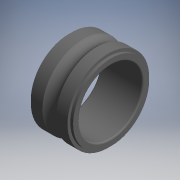
# Autodesk Inventor part: MR126ZZ Inner Ring
Saved by Autodesk Inventor 2017.3 (Build 213256000, 256)
## iProperties
Part Number: MR126ZZ Inner Ring
Material: Generic
Catalog Web Link: www.cadenas.de
Description: shielde_type_zz_zzs_IR-
Vendor: NSK_RB
Document SubType Name: Modeling
Designer: partserver
Manufacturer: NSK_RB
Mass: 0.0656368 g
Surface Area: 2.08449 cm^2
Volume: 0.0656368 cm^3
Density: 1 g/cm^3
Appearance: PSOLRGB-128-128-128
Category: PARTsolutions
Company: NSK_RB
Title: MR126ZZ Inner Ring
Author: Cadenas PARTsolutions
PSOL_IDENT_0: {$CADENAS_DATA\23d-libs\nsk_rb\roller_bearings\deep_groove_bb\exstra_small_miniatur_bb\metric_design
PSOL_IDENT_1: \shielded_type_zz_zzs_ir.prj},193 {VTYP=3D},{NB=MR126ZZ Inner Ring},{LINA=MR126ZZ Inner Ring},{NN=sh
PSOL_IDENT_2: ielde_type_zz_zzs_IR},{DATE=16.07.2021 00:25:30},{GEOMDATE=04.01.2008 00:00:00},{VERSION=},{LINEID=5
PSOL_IDENT_3: 90},{WBVAR=},{WBNUMERIC=}  {NB=MR126ZZ Inner Ring},{LINA=MR126ZZ Inner Ring},{KT=DUMMY},{IDNR=},{STA
PSOL_IDENT_4: N=Standard},{ORDER=MR126ZZ},{SD=6.0},{X=6.0},{DI1=7.73},{DI2=7.20},{SDE1=10.19},{SDE2=10.90},{D=12},
PSOL_IDENT_5: {DD=12},{B=0.0},{B1=4.0},{R=0.00},{R1=0.15},{CR1=715},{COR1=292},{CR2=73},{COR2=30.0},{LG=43000},{LO=
PSOL_IDENT_6: 50000},{DA=0.0},{DB=7.2},{DA1=0.0},{DB1=10.9},{RA=0.00},{RB=0.15},{MASS=1.74},{SC=1},{N=12}
NB: MR126ZZ Inner Ring
NN: shielde_type_zz_zzs_IR
NBSYN: $ORDER. Inner Ring
LINA: MR126ZZ Inner Ring
CATALOG: NSK Rolling Bearing
STAN: Standard
ORDER: MR126ZZ
SD: 6
X: 6
DI1: 7.73
DI2: 7.2
SDE1: 10.19
SDE2: 10.9
D: 12
DD: 12
B: 0
B1: 4
R: 0
R1: 0.15
CR1: 715
COR1: 292
CR2: 73
COR2: 30
LG: 43000
LO: 50000
DA: 0
DB: 7.2
DA1: 0
DB1: 10.9
RA: 0
RB: 0.15
MASS: 1.74
SC: 1
SUPPLIER: NSK_RB
ARTICLENO: MR126ZZ Inner Ring
BOMINFO: MR126ZZ Inner Ring
CREATOR: CADENAS GmbH
Autodesk Inventor part; units mm, degrees
sketch "Sketch_2" plane through (0, 0, 0) normal (0, 0, 1) x (1, 0, 0)
  line L0 (4, 0) -> (0, 0)
  arc A0 (0, 3.15) -> (0.15, 3) centre (0.15, 3.15) ccw
  line L1 (0.15, 3) -> (3.85, 3)
  arc A1 (3.85, 3) -> (4, 3.15) centre (3.85, 3.15) ccw
  line L2 (4, 3.15) -> (4, 3.6)
  line L3 (4, 3.6) -> (3.7344, 3.6)
  line L4 (3.7344, 3.6) -> (3.7344, 3.865)
  line L5 (3.7344, 3.865) -> (2.6378, 3.865)
  arc A2 (1.3622, 3.865) -> (2.6378, 3.865) centre (2, 4.5) ccw
  line L6 (1.3622, 3.865) -> (0.2656, 3.865)
  line L7 (0.2656, 3.865) -> (0.2656, 3.6)
  line L8 (0.2656, 3.6) -> (0, 3.6)
  line L9 (0, 3.6) -> (0, 3.15)
  constraints: 20 end point, 6 point on circle, 3 centre point
revolve "Revolution1" add sketch "Sketch_2" angle 360 about axis through (4, 0, 0) along (1, 0, 0)
ref_plane "ip_st_ir_1_1_XY" through (2, 4.5, 0) normal (1, 0, 0) x (0, 0, -1)
ref_plane "ip_st_ir_1_1_YZ" through (2, 4.5, 0) normal (0, 0, -1) x (0, 1, 0)
ref_plane "ip_st_ir_1_1_ZX" through (2, 4.5, 0) normal (0, 1, 0) x (1, 0, 0)
ref_plane "ip_st_ir_1_10_XY" through (2, 0, -4.5) normal (1, 0, 0) x (0, 0, -1)
ref_plane "ip_st_ir_1_10_YZ" through (2, 0, -4.5) normal (0, 0, -1) x (0, 1, 0)
ref_plane "ip_st_ir_1_10_ZX" through (2, 0, -4.5) normal (0, 1, 0) x (1, 0, 0)
ref_plane "ip_st_ir_1_11_XY" through (2, 2.25, -3.8971) normal (1, 0, 0) x (0, 0, -1)
ref_plane "ip_st_ir_1_11_YZ" through (2, 2.25, -3.8971) normal (0, 0, -1) x (0, 1, 0)
ref_plane "ip_st_ir_1_11_ZX" through (2, 2.25, -3.8971) normal (0, 1, 0) x (1, 0, 0)
ref_plane "ip_st_ir_1_12_XY" through (2, 3.8971, -2.25) normal (1, 0, 0) x (0, 0, -1)
ref_plane "ip_st_ir_1_12_YZ" through (2, 3.8971, -2.25) normal (0, 0, -1) x (0, 1, 0)
ref_plane "ip_st_ir_1_12_ZX" through (2, 3.8971, -2.25) normal (0, 1, 0) x (1, 0, 0)
ref_plane "ip_st_ir_1_2_XY" through (2, 3.8971, 2.25) normal (1, 0, 0) x (0, 0, -1)
ref_plane "ip_st_ir_1_2_YZ" through (2, 3.8971, 2.25) normal (0, 0, -1) x (0, 1, 0)
ref_plane "ip_st_ir_1_2_ZX" through (2, 3.8971, 2.25) normal (0, 1, 0) x (1, 0, 0)
ref_plane "ip_st_ir_1_3_XY" through (2, 2.25, 3.8971) normal (1, 0, 0) x (0, 0, -1)
ref_plane "ip_st_ir_1_3_YZ" through (2, 2.25, 3.8971) normal (0, 0, -1) x (0, 1, 0)
ref_plane "ip_st_ir_1_3_ZX" through (2, 2.25, 3.8971) normal (0, 1, 0) x (1, 0, 0)
ref_plane "ip_st_ir_1_4_XY" through (2, 0, 4.5) normal (1, 0, 0) x (0, 0, -1)
ref_plane "ip_st_ir_1_4_YZ" through (2, 0, 4.5) normal (0, 0, -1) x (0, 1, 0)
ref_plane "ip_st_ir_1_4_ZX" through (2, 0, 4.5) normal (0, 1, 0) x (1, 0, 0)
ref_plane "ip_st_ir_1_5_XY" through (2, -2.25, 3.8971) normal (1, 0, 0) x (0, 0, -1)
ref_plane "ip_st_ir_1_5_YZ" through (2, -2.25, 3.8971) normal (0, 0, -1) x (0, 1, 0)
ref_plane "ip_st_ir_1_5_ZX" through (2, -2.25, 3.8971) normal (0, 1, 0) x (1, 0, 0)
ref_plane "ip_st_ir_1_6_XY" through (2, -3.8971, 2.25) normal (1, 0, 0) x (0, 0, -1)
ref_plane "ip_st_ir_1_6_YZ" through (2, -3.8971, 2.25) normal (0, 0, -1) x (0, 1, 0)
ref_plane "ip_st_ir_1_6_ZX" through (2, -3.8971, 2.25) normal (0, 1, 0) x (1, 0, 0)
ref_plane "ip_st_ir_1_7_XY" through (2, -4.5, 0) normal (1, 0, 0) x (0, 0, -1)
ref_plane "ip_st_ir_1_7_YZ" through (2, -4.5, 0) normal (0, 0, -1) x (0, 1, 0)
ref_plane "ip_st_ir_1_7_ZX" through (2, -4.5, 0) normal (0, 1, 0) x (1, 0, 0)
ref_plane "ip_st_ir_1_8_XY" through (2, -3.8971, -2.25) normal (1, 0, 0) x (0, 0, -1)
ref_plane "ip_st_ir_1_8_YZ" through (2, -3.8971, -2.25) normal (0, 0, -1) x (0, 1, 0)
ref_plane "ip_st_ir_1_8_ZX" through (2, -3.8971, -2.25) normal (0, 1, 0) x (1, 0, 0)
ref_plane "ip_st_ir_1_9_XY" through (2, -2.25, -3.8971) normal (1, 0, 0) x (0, 0, -1)
ref_plane "ip_st_ir_1_9_YZ" through (2, -2.25, -3.8971) normal (0, 0, -1) x (0, 1, 0)
ref_plane "ip_st_ir_1_9_ZX" through (2, -2.25, -3.8971) normal (0, 1, 0) x (1, 0, 0)
ref_plane "ip_st_ir_1a_XY" through (0, 0, 0) normal (1, 0, 0) x (0, 0, -1)
ref_plane "ip_st_ir_1a_YZ" through (0, 0, 0) normal (0, 0, -1) x (0, 1, 0)
ref_plane "ip_st_ir_1a_ZX" through (0, 0, 0) normal (0, 1, 0) x (1, 0, 0)
ref_plane "ip_st_ir_2a_XY" through (0.2656, 0, 0) normal (1, 0, 0) x (0, 0, -1)
ref_plane "ip_st_ir_2a_YZ" through (0.2656, 0, 0) normal (0, 0, -1) x (0, 1, 0)
ref_plane "ip_st_ir_2a_ZX" through (0.2656, 0, 0) normal (0, 1, 0) x (1, 0, 0)
body "Solid1"
